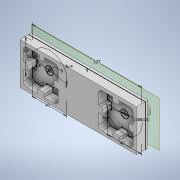
# Autodesk Inventor part: Stellager_adapter
Saved by Autodesk Inventor 2022 (Build 260153000, 153)
## iProperties
Created: 2023-06-27
Part Number: Stellager_adapter
Material: Generisch
Document SubType Name: Modeling
Designer: aewalder
Density: 1 g/cm^3
Appearance: Vorgabe
Author: aewalder
Autodesk Inventor part; units mm, degrees
ref_plane "YZ Plane" through (0, 0, 0) normal (1, 0, 0) x (0, 1, 0)
ref_plane "XZ Plane" through (0, 0, 0) normal (0, 1, 0) x (-1, 0, 0)
ref_plane "XY Plane" through (0, 0, 0) normal (0, 0, 1) x (1, 0, 0)
sketch "Sketch1" plane through (0, 0, 0) normal (0, 0, 1) x (1, 0, 0)
  line L0 (-63.5, 20) -> (63.5, 20)
  line L1 (63.5, 20) -> (63.5, -20)
  line L2 (63.5, -20) -> (-63.5, -20)
  line L3 (-63.5, -20) -> (-63.5, 20)
  line L4 (-63.5, 20) -> (63.5, -20) construction
  line L5 (63.5, 20) -> (-63.5, -20) construction
  line L6 (-63.5, 3.9) -> (-58.5, 3.9)
  line L7 (-58.5, 3.9) -> (-58.5, -3.9)
  line L8 (-58.5, -3.9) -> (-63.5, -3.9)
  line L9 (-63.5, -3.9) -> (-63.5, 3.9)
  line L10 (0, 20) -> (0, -20) construction
  line L11 (63.5, 3.9) -> (58.5, 3.9)
  line L12 (58.5, 3.9) -> (58.5, -3.9)
  line L13 (58.5, -3.9) -> (63.5, -3.9)
  line L14 (63.5, -3.9) -> (63.5, 3.9)
  line L15 (-63.5, 20) -> (-23.5, 20) construction
  line L16 (-23.5, 20) -> (-23.5, -20)
  line L17 (-23.5, -20) -> (-63.5, -20) construction
  line L18 (-63.5, -20) -> (-63.5, 20) construction
  line L19 (-63.5, 0) -> (-23.5, 0) construction
  line L20 (63.5, 20) -> (23.5, 20) construction
  line L21 (23.5, 20) -> (23.5, -20)
  line L22 (23.5, -20) -> (63.5, -20) construction
  line L23 (63.5, -20) -> (63.5, 20) construction
  line L24 (23.5, 0) -> (63.5, 0) construction
  line L25 (-47.4, -20) -> (-47.4, -15)
  line L26 (-47.4, -15) -> (-39.6, -15)
  line L27 (-39.6, -20) -> (-47.4, -20)
  line L28 (-39.6, -15) -> (-39.6, -20)
  line L29 (-23.5, -3.9) -> (-28.5, -3.9)
  line L30 (-28.5, -3.9) -> (-28.5, 3.9)
  line L31 (-23.5, 3.9) -> (-23.5, -3.9)
  line L32 (-28.5, 3.9) -> (-23.5, 3.9)
  line L33 (-39.6, 20) -> (-39.6, 15)
  line L34 (-39.6, 15) -> (-47.4, 15)
  line L35 (-47.4, 20) -> (-39.6, 20)
  line L36 (-47.4, 15) -> (-47.4, 20)
  line L37 (39.6, 20) -> (39.6, 15)
  line L38 (39.6, 15) -> (47.4, 15)
  line L39 (47.4, 15) -> (47.4, 20)
  line L40 (47.4, 20) -> (39.6, 20)
  line L41 (23.5, -3.9) -> (28.5, -3.9)
  line L42 (28.5, -3.9) -> (28.5, 3.9)
  line L43 (28.5, 3.9) -> (23.5, 3.9)
  line L44 (23.5, 3.9) -> (23.5, -3.9)
  line L45 (47.4, -20) -> (47.4, -15)
  line L46 (47.4, -15) -> (39.6, -15)
  line L47 (39.6, -15) -> (39.6, -20)
  line L48 (39.6, -20) -> (47.4, -20)
  line L49 (67.5, 24) -> (-67.5, 24)
  line L50 (-67.5, 24) -> (-67.5, -24)
  line L51 (-67.5, -24) -> (67.5, -24)
  line L52 (67.5, -24) -> (67.5, 24)
  line L53 (-19.5, 24) -> (-19.5, -24)
  line L54 (19.5, 24) -> (19.5, -24)
  circle A0 centre (-43.5, 0) radius 4.5
  circle A1 centre (43.5, 0) radius 4.5
  point P0 (0, 0)
  point P1 (-43.5, -20)
  point P2 (-23.5, 0)
  point P3 (-43.5, 20)
  point P4 (43.5, 20)
  point P5 (23.5, 0)
  point P6 (43.5, -20)
  dimension "d0" = 127
  dimension "d1" = 40
  dimension "d2" = 7.8
  dimension "d3" = 5
  dimension "d4" = 40
  dimension "d5" = 40
  dimension "d8" = 360
  dimension "d12" = 360
  dimension "d14" = 4
  dimension "d15" = 4
  dimension "d16" = 4
  dimension "d21" = 9
  dimension "d22" = 9
  constraints: 110 end point, 10 midpoint, 10 parallel, 7 perpendicular, 7 point on line, 5 horizontal, 5 symmetric about line, 2 centre point, 2 coincident, 77 other
  measures "d0" distance of L0.start L0.end
  measures "d1" distance of L2.end L0.start
  measures "d2" distance of L6.end L7.end
  measures "d3" distance of L7.end L8.end
  measures "d4" distance between parallel lines of L18 L16
  measures "d5" distance between parallel lines of L1 L21
  measures "d14" distance between parallel lines of L0 L49
  measures "d15" distance between parallel lines of L21 L54
  measures "d16" distance between parallel lines of L53 L16
  measures "d21" diameter of A0
  measures "d22" diameter of A1
extrude "Extrusion1" add sketch "Sketch1" along normal blind 10 contours L3 L2 L53 L51 L50 L49 L0 | L0 L33 L34 L36 | L6 L7 L8 L3 | L0 L53 L2 L16 | L16 L29 L30 L32 | L25 L26 L28 L2 | L54 L49 L52 L51 L2 L1 L0 | L0 L21 L2 L54 | L0 L39 L38 L37 | L43 L42 L41 L21 | L47 L46 L45 L2 | L1 L13 L12 L11
extrude "Extrusion2" add sketch "Sketch1" against normal blind 3
ref_plane "Work Plane1" through (0, 0, -9.5) normal (0, 0, -1) x (-1, 0, 0)
sketch "Sketch2" plane through (0, 0, -9.5) normal (0, 0, -1) x (-1, 0, 0)
  line L0 (-50.5, 0) -> (-44.5, 0) construction
  line L1 (-50.5, -6.5) -> (-44.5, -6.5)
  line L2 (-44.5, 6.5) -> (-50.5, 6.5)
  arc A0 (-50.5, 6.5) -> (-50.5, -6.5) centre (-50.5, 0) ccw
  arc A1 (-44.5, -6.5) -> (-44.5, 6.5) centre (-44.5, 0) ccw
  line L3 (19.5, -24) -> (-19.5, -24) construction
  line L4 (0, -24) -> (0, 24) construction
  line L5 (-19.5, 24) -> (19.5, 24) construction
  line L6 (0, 0) -> (-67.5, 0) construction
  line L7 (-67.5, -24) -> (-67.5, 24) construction
  line L8 (50.5, 0) -> (44.5, 0) construction
  line L9 (50.5, -6.5) -> (44.5, -6.5)
  line L10 (44.5, 6.5) -> (50.5, 6.5)
  arc A2 (50.5, -6.5) -> (50.5, 6.5) centre (50.5, 0) ccw
  arc A3 (44.5, 6.5) -> (44.5, -6.5) centre (44.5, 0) ccw
  point P0 (-47.5, 0)
  point P1 (47.5, 0)
  dimension "d24" = 44.5
  dimension "d25" = 13
  dimension "d26" = 6
  constraints: 20 end point, 8 point on circle, 7 symmetric about line, 4 centre point, 4 midpoint, 4 tangent, 1 collinear, 1 horizontal, 1 parallel, 2 other
  measures "d24" distance from line of L4 L0.end
  measures "d25" distance between parallel lines of L2 L1
  measures "d26" distance of L0.start L0.end
sketch "Sketch3" plane through (0, 0, -3) normal (0, 0, -1) x (-1, 0, 0)
  line L0 (-56.95, 0) -> (-38, 0) construction
  line L1 (-56.95, -6.5) -> (-38, -6.5)
  line L2 (-38, 6.5) -> (-56.95, 6.5)
  arc A0 (-56.95, 6.5) -> (-56.95, -6.5) centre (-56.95, 0) ccw
  arc A1 (-38, -6.5) -> (-38, 6.5) centre (-38, 0) ccw
  line L3 (0, -24) -> (0, 24) construction
  line L4 (0, 0) -> (-67.5, 0) construction
  line L5 (56.95, 0) -> (38, 0) construction
  line L6 (56.95, -6.5) -> (38, -6.5)
  line L7 (38, 6.5) -> (56.95, 6.5)
  arc A2 (56.95, -6.5) -> (56.95, 6.5) centre (56.95, 0) ccw
  arc A3 (38, 6.5) -> (38, -6.5) centre (38, 0) ccw
  point P0 (-47.475, 0)
  point P1 (47.475, 0)
  dimension "d27" = 18.95
  dimension "d28" = 13
  dimension "d29" = 38
  constraints: 16 end point, 8 point on circle, 7 symmetric about line, 4 centre point, 4 tangent, 1 collinear, 1 horizontal, 1 midpoint, 1 parallel, 2 other
  measures "d27" distance of L0.start L0.end
  measures "d28" distance between parallel lines of L2 L1
  measures "d29" distance from line of L3 L0.end
extrude "Extrusion3" add sketch "Sketch3" along normal up to surface (6.5 mm away)
extrude "Extrusion4" add sketch "Sketch2" along normal blind 7.5
delete faces "Delete Face1" heal yes whole lump no faces at (-40.9932, 1.1627, -3) (46.0068, 1.1627, -3)
fillet "Fillet1" radius 4 8 edges at (-23.5, 20, 5) (-63.5, 20, 5) (-23.5, -20, 5) (-63.5, -20, 5) (23.5, -20, 5) (63.5, -20, 5) (63.5, 20, 5) (23.5, 20, 5)
fillet "Fillet2" radius 2 16 edges at (28.5, -3.9, 5) (28.5, 3.9, 5) (39.6, 15, 5) (47.4, 15, 5) (47.4, -15, 5) (58.5, -3.9, 5) (58.5, 3.9, 5) (39.6, -15, 5) (-47.4, -15, 5) (-39.6, -15, 5) (-58.5, -3.9, 5) (-58.5, 3.9, 5) (-39.6, 15, 5) (-28.5, 3.9, 5) (-28.5, -3.9, 5) (-47.4, 15, 5)
sketch "Sketch4" plane through (-38, -6.5, -9.5) normal (0, 0, -1) x (-1, 0, 0)
  arc A0 (12.5, 0) -> (12.5, 13) centre (12.5, 6.5) ccw construction
  line L0 (12.5, 0) -> (12.5, 13) construction
  line L1 (0, 13) -> (18.95, 13) construction
  line L2 (12.5, 13) -> (12.5, 0) construction
  line L3 (18.95, 0) -> (0, 0) construction
  arc A1 (12.5, 0) -> (12.5, 13) centre (12.5, 6.5) ccw
  line L4 (18.95, 0) -> (0, 0) projected
  arc A2 (18.95, 0) -> (18.95, 13) centre (18.95, 6.5) ccw projected
  line L5 (0, 13) -> (18.95, 13) projected
  line L6 (29.5, 30.5) -> (-105.5, 30.5) construction
  line L7 (-38, 30.5) -> (-38, -17.5) construction
  line L8 (-105.5, -17.5) -> (29.5, -17.5) construction
  arc A3 (-88.5, 13) -> (-88.5, 0) centre (-88.5, 6.5) ccw
  line L9 (-76, 0) -> (-94.95, 0) projected
  arc A4 (-94.95, 13) -> (-94.95, 0) centre (-94.95, 6.5) ccw projected
  line L10 (-94.95, 13) -> (-76, 13) projected
  point P0 (-38, 6.5)
  constraints: 6 end point, 4 point on circle, 3 symmetric about line, 2 centre point, 2 midpoint, 2 point on line, 2 vertical, 1 concentric, 1 other
sketch "Sketch5" plane through (0, 0, 0) normal (0, 0, 1) x (1, 0, 0)
  line L0 (19.5, 24) -> (19.5, -24) projected
  line L1 (19.5, 24) -> (-19.5, 24) projected
  line L2 (-19.5, -24) -> (-19.5, 24) projected
  line L3 (-19.5, -24) -> (19.5, -24) projected
  point P0 (0, 0)
extrude "Extrusion5" add sketch "Sketch5" along normal up to surface (10 mm away)
extrude "Extrusion6" cut sketch "Sketch4" against normal up to surface (6.5 mm away)
thicken "Thicken1" operation add thickness 0.15 both sides no extend neighbours yes toward (0, 1, 0) faces at (-35.5667, 20, 3.3333) (-24.195, 18.2533, 3.3333) (-23.5, 11.9667, 3.3333) (-24.5, 3.9, 3.3333) (-27.8603, 3.3661, 3.3333) (-28.5, 0.6333, 3.3333) (-27.9661, -3.2603, 3.3333) (-25.5, -3.9, 3.3333) (-23.5, -7.9333, 3.3333) (-23.6777, -17.179, 3.3333) (-31.5333, -20, 3.3333) (-39.6, 18, 3.3333) (-41.3019, 15.0223, 3.3333) (-44.1333, 15, 6.6667) (-46.8661, 15.6397, 3.3333) (-47.4, 19, 3.3333) (-55.4667, 20, 3.3333) (-62.2207, 18.9322, 3.3333) (-63.5, 7.9333, 3.3333) (-61.5, 3.9, 3.3333) (-58.7679, 2.9, 3.3333) (-58.5, -0.6333, 3.3333) (-58.7679, -2.9, 3.3333) (-62.5, -3.9, 3.3333) (-63.5, -11.9667, 3.3333) (-62.2207, -18.9322, 3.3333) (-51.4333, -20, 3.3333) (-47.4, -18, 3.3333) (-46.4, -15.2679, 3.3333) (-42.8667, -15, 3.3333) (-40.6, -15.2679, 3.3333) (-39.6, -19, 3.3333) (35.5667, -20, 3.3333) (24.7793, -18.9322, 3.3333) (23.5, -11.9667, 3.3333) (44.1333, -15, 3.3333) (39.6223, -16.7019, 3.3333) (46.4, -15.2679, 3.3333) (39.6, -18, 3.3333) (47.4, -19, 3.3333) (55.4667, -20, 3.3333) (62.2207, -18.9322, 3.3333) (63.5, -7.9333, 3.3333) (58.7679, 2.9, 3.3333) (62.5, 3.9, 3.3333) (58.5, 0.6333, 3.3333) (58.7679, -2.9, 3.3333) (61.5, -3.9, 3.3333) (63.5, 11.9667, 6.6667) (62.4322, 18.7207, 3.3333) (51.4333, 20, 3.3333) (42.8667, 15, 3.3333) (46.8661, 15.6397, 3.3333) (41.3019, 15.0223, 3.3333) (47.4, 18, 3.3333) (39.6, 19, 3.3333) (31.5333, 20, 3.3333) (24.0359, 18, 3.3333) (23.5, 7.9333, 3.3333) (25.5, 3.9, 3.3333) (27.0895, 3.8111, 3.3333) (28.5, -0.6333, 3.3333) (27.6266, -3.5525, 3.3333) (24.5, -3.9, 3.3333)
equation "\"d15\" = d14"
equation "\"d16\" = d14"
body "Solid1"
